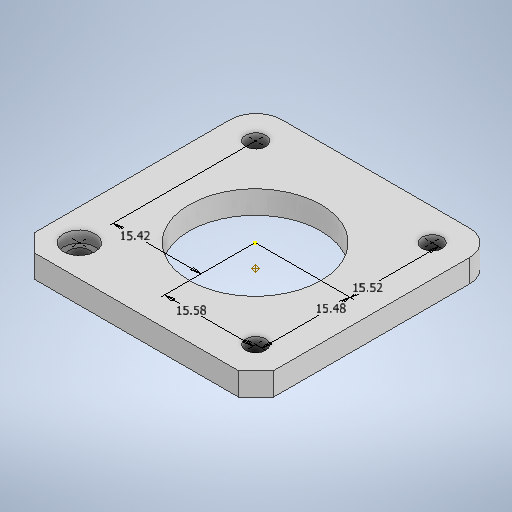
# Autodesk Inventor part: Extruder Housing
Saved by Autodesk Inventor 2025 (Build 290162000, 162)
## iProperties
Created: 2025-03-12
Part Number: Extruder Housing
Material: Generic
Document SubType Name: Modeling
Designer: MAL16204
Density: 1 g/cm^3
Appearance: Default
Author: MAL16204
Autodesk Inventor part; units mm, degrees
ref_plane "YZ Plane" through (0, 0, 0) normal (1, 0, 0) x (0, 1, 0)
ref_plane "XZ Plane" through (0, 0, 0) normal (0, 1, 0) x (-1, 0, 0)
ref_plane "XY Plane" through (0, 0, 0) normal (0, 0, 1) x (1, 0, 0)
sketch "Sketch1" plane through (0, 0, 0) normal (0, 1, 0) x (-1, 0, 0)
  circle A0 centre (0, 0) radius 11.56
  line L0 (20.9, -21.04) -> (-21.11, -21.04)
  line L1 (20.9, 20.96) -> (-21.11, 20.96)
  line L2 (20.9, 20.96) -> (20.9, -21.04)
  line L3 (-21.11, 20.96) -> (-21.11, -21.04)
  dimension "d1" = 23.12
  dimension "d2" = 21.04
  dimension "d3" = 20.9
  dimension "d4" = 20.96
  dimension "d5" = 21.11
  constraints: 8 end point, 2 horizontal, 2 vertical, 1 centre point, 1 coincident
  measures "d1" diameter of A0
  measures "d2" distance from line of A0.centre L0
  measures "d3" distance from line of L2 A0.centre
  measures "d4" distance from line of L1 A0.centre
  measures "d5" distance from line of L3 A0.centre
extrude "Extrusion1" add sketch "Sketch1" along normal blind 4.02
sketch "Sketch2" plane through (0, 4.02, 0) normal (0, 1, 0) x (1, 0, 0)
  point P0 (0, 0)
  point P1 (15.58, -15.48)
  point P2 (15.58, 15.52)
  point P3 (-15.42, 15.52)
  point P4 (-15.42, -15.48)
  dimension "d8" = 15.52
  dimension "d9" = 15.48
  dimension "d10" = 15.42
  dimension "d11" = 15.58
  constraints: 2 horizontal alignment, 2 vertical alignment
  measures "d8" vertical distance of point (0, 0) point (15.58, 15.52)
  measures "d9" vertical distance of point (0, 0) point (15.58, -15.48)
  measures "d10" horizontal distance of point (0, 0) point (-15.42, 15.52)
  measures "d11" horizontal distance of point (0, 0) point (15.58, -15.48)
hole "Hole1" at (15.58, 4.02, 15.48) at (15.58, 4.02, -15.52) at (-15.42, 4.02, -15.52) direction (0, -1, 0) diameter 3.52 end through all
hole "Hole2" at (-15.42, 4.02, 15.48) direction (0, -1, 0) diameter 3.52 end through all counterbore diameter 5.52 counterbore depth 2
fillet "Fillet1" radius 4.5 2 edges at (-20.9, 2.01, -21.04) (21.11, 2.01, -21.04)
chamfer "Chamfer1" distance 3 angle 45 2 edges at (-20.9, 2.01, 20.96) (21.11, 2.01, 20.96)
body "Solid1"
